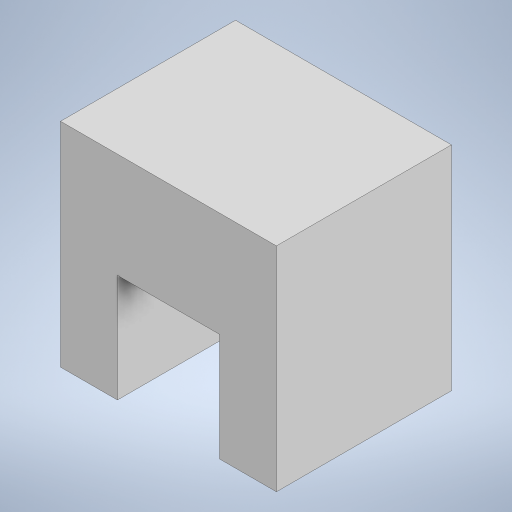
# Autodesk Inventor part: Socket
Saved by Autodesk Inventor 2024.3 (Build 283343000, 343)
## iProperties
Created: 2025-01-23
Part Number: Socket
Material: Generic
Document SubType Name: Modeling
Designer: ASUS TUF
Density: 1 g/cm^3
Appearance: Default
Author: ASUS TUF
Autodesk Inventor part; units mm, degrees
ref_plane "YZ Plane" through (0, 0, 0) normal (1, 0, 0) x (0, 1, 0)
ref_plane "XZ Plane" through (0, 0, 0) normal (0, 1, 0) x (-1, 0, 0)
ref_plane "XY Plane" through (0, 0, 0) normal (0, 0, 1) x (1, 0, 0)
sketch "Sketch1" plane through (0, 0, 0) normal (0, 0, 1) x (1, 0, 0)
  line L0 (-3.7, -3.65) -> (3.7, -3.65)
  line L1 (3.7, -3.65) -> (3.7, 3.65)
  line L2 (3.7, 3.65) -> (-3.7, 3.65)
  line L3 (-3.7, 3.65) -> (-3.7, -3.65)
  line L4 (-3.7, -3.65) -> (3.7, 3.65) construction
  line L5 (3.7, -3.65) -> (-3.7, 3.65) construction
  line L6 (-1.75, -3.65) -> (1.75, -3.65)
  line L7 (1.75, -3.65) -> (1.75, 0.05)
  line L8 (1.75, 0.05) -> (-1.75, 0.05)
  line L9 (-1.75, 0.05) -> (-1.75, -3.65)
  point P0 (0, 0)
  point P1 (0, 0.05)
  dimension "d0" = 7.4
  dimension "d1" = 7.3
  dimension "d2" = 3.5
  dimension "d3" = 3.7
  constraints: 20 end point, 4 parallel, 3 midpoint, 2 horizontal, 2 perpendicular, 1 point on line, 1 vertical alignment
  measures "d0" distance of L2.end L1.end
  measures "d1" distance of L1.end L0.end
  measures "d2" distance of L8.end L7.end
  measures "d3" distance of L7.end L6.end
extrude "Extrusion1" add sketch "Sketch1" along normal blind 6 contours L3 L2 L1 L0 L7 L8 L9
extrude "Extrusion2" add sketch "Sketch1" along normal blind 2 contours L9 L8 L7 L0
body "Solid1"
